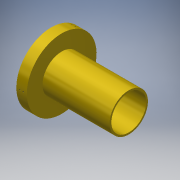
# Autodesk Inventor part: ALPHA_001157_EndNosePiece
Saved by Autodesk Inventor 2017 (Build 210142000, 142)
## iProperties
Created: 2015-11-18
Part Number: ALPHA_001157_EndNosePiece
Material: Generic
Document SubType Name: Modeling
Designer: massen
Density: 1 g/cm^3
Appearance: Glossy - Gold
Author: massen
Autodesk Inventor part; units mm, degrees
ref_plane "YZ Plane" through (0, 0, 0) normal (1, 0, 0) x (0, 1, 0)
ref_plane "XZ Plane" through (0, 0, 0) normal (0, 1, 0) x (-1, 0, 0)
sketch "Sketch1" plane through (0, 0, 0) normal (0, 0, 1) x (1, 0, 0)
  line L0 (-44.5, 40) -> (-32.5, 40)
  line L1 (-32.5, 40) -> (-32.5, 22)
  line L2 (-32.5, 22) -> (44.5, 22)
  line L3 (44.5, 22) -> (44.5, 20)
  line L4 (44.5, 20) -> (-44.5, 20)
  line L5 (-44.5, 20) -> (-44.5, 40)
  line L6 (-62.3, 0) -> (62.3, 0) projected
  point P0 (0, 0)
  point P1 (0, 20)
  dimension "d0" = 12
  dimension "d1" = 89
  dimension "d2" = 40
  dimension "d3" = 44
  dimension "d4" = 80
  constraints: 12 end point, 4 parallel, 1 horizontal, 1 midpoint, 1 perpendicular, 1 vertical alignment
  measures "d0" distance between parallel lines of L5 L1
  measures "d1" distance between parallel lines of L3 L5
  measures "d2" diameter of L4 L6
  measures "d3" diameter of L2 L6
  measures "d4" diameter of L0 L6
revolve "Revolution1" add sketch "Sketch1" angle 360 about axis through (-10, 0, 0) along (1, 0, 0)
ref_plane "Work Plane1" through (-38.5, 0, 40) normal (0, 0, 1) x (1, 0, 0)
sketch "Sketch2" plane through (-38.5, 0, 40) normal (0, 0, 1) x (1, 0, 0)
  line L0 (-2, 0) -> (2, 0) construction
  line L1 (-6, -40) -> (-6, 40) projected
  line L2 (6, -40) -> (6, 40) projected
  line L3 (-6, 0) -> (6, 0) construction
  point P0 (38.5, 0)
  point P1 (0, 0)
  dimension "d6" = 4
  constraints: 4 end point, 4 midpoint, 2 coincident, 1 horizontal
  measures "d6" distance of L0.start L0.end
hole "Hole1" at (-40.5, 0, 40) at (-36.5, 0, 40) direction (0, 0, -1) diameter 1.567 depth 8 tip angle 118 thread size "M2x0.4" class "6H" standard "ISO Metric profile"
pattern_circular "Circular Pattern1" count 3 over 360 about axis through (0, 0, 0) along (1, 0, 0) of "Hole1"
body "Solid1"
